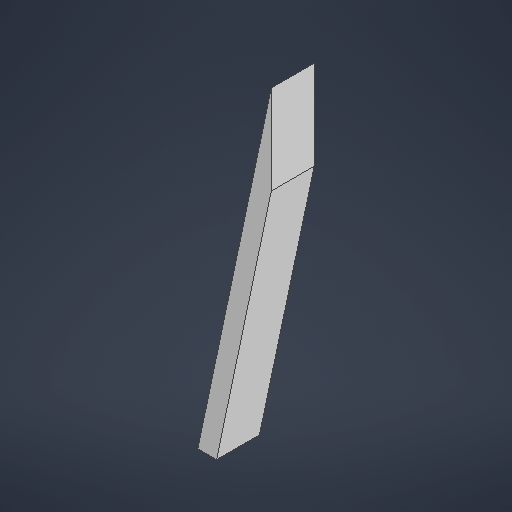
# Autodesk Inventor part: S_2x4x29.334
Saved by Autodesk Inventor 2026 (Build 300175000, 175)
## iProperties
Created: 2025-09-08
Part Number: S_2x4x29.334
Material: Generic
Document SubType Name: Modeling
Designer: trott
Density: 1 g/cm^3
Appearance: Default
Author: trott
Autodesk Inventor part; units mm, degrees
ref_plane "YZ Plane" through (0, 0, 0) normal (1, 0, 0) x (0, 1, 0)
ref_plane "XZ Plane" through (0, 0, 0) normal (0, 1, 0) x (-1, 0, 0)
ref_plane "XY Plane" through (0, 0, 0) normal (0, 0, 1) x (1, 0, 0)
sketch "Sketch1" plane through (0, 0, 0) normal (0, 0, 1) x (1, 0, 0)
  line L0 (0, 0) -> (1219.2, 0)
  line L1 (0, 0) -> (152.4, 0)
  line L2 (152.4, 0) -> (152.4, 762)
  line L3 (152.4, 762) -> (1066.8, 762)
  line L4 (1066.8, 762) -> (1066.8, 0)
  line L5 (152.4, 762) -> (152.4, 723.9)
  line L6 (152.4, 723.9) -> (1066.8, 723.9)
  line L7 (152.4, 0) -> (152.4, 38.1)
  line L8 (152.4, 38.1) -> (1066.8, 38.1)
  line L9 (1066.8, 38.1) -> (1219.2, 38.1)
  line L10 (1219.2, 38.1) -> (1219.2, 0)
  line L11 (152.4, 38.1) -> (0, 38.1)
  line L12 (0, 38.1) -> (0, 0)
  line L13 (0, 38.1) -> (152.4, 762)
  line L14 (1219.2, 38.1) -> (1066.8, 762)
  line L15 (0, 38.1) -> (37.2827, 30.251)
  line L16 (152.4, 762) -> (189.6827, 754.151)
  line L17 (189.6827, 754.151) -> (37.2827, 30.251)
  point P0 (38.9352, 38.1)
  point P1 (152.4, 577.058)
  dimension "d0" = 1219.2
  dimension "d1" = 152.4
  dimension "d2" = 762
  dimension "d3" = 914.4
  dimension "d4" = 38.1
  dimension "d5" = 38.1
  dimension "d6" = 38.1
  dimension "d7" = 38.1
  constraints: 36 end point, 8 perpendicular, 7 point on line, 3 horizontal
  measures "d0" distance of L0.start L0.end
  measures "d1" distance of L0.start L1.end
  measures "d2" distance of L1.end L2.end
  measures "d3" distance of L2.end L3.end
  measures "d4" distance of L2.end L5.end
  measures "d5" distance of L1.end L7.end
  measures "d6" distance of L11.end L15.end
  measures "d7" distance of L2.end L16.end
extrude "Extrusion1" add sketch "Sketch1" along normal blind 88.9 contours L13 L2 L17 L11
body "Solid1"
